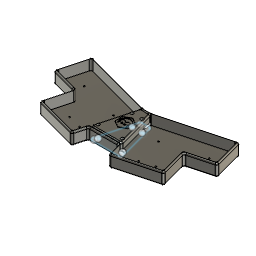
rattlemebonez32 v7 (Autodesk Fusion 360 design; units mm, degrees)
Autodesk Fusion 360 part; units mm, degrees
sketch "complete_combo(6)" plane through (0, 0, 0) normal (0, 0, 1) x (1, 0, 0)
  line L0 (-3.352867, 24.192112) -> (4.411704, 53.169887)
  line L1 (6.861194, 54.5841) -> (80.98315, 34.723182)
  line L2 (81.500788, 34.655034) -> (87.939454, 34.655034)
  line L3 (88.457092, 34.723182) -> (162.579048, 54.5841)
  line L4 (165.028537, 53.169887) -> (172.793109, 24.192112)
  line L5 (171.378895, 21.742622) -> (146.264824, 15.013327)
  line L6 (144.85061, 12.563837) -> (151.579905, -12.550234)
  line L7 (150.165692, -14.999724) -> (106.699029, -26.646581)
  line L8 (104.24954, -25.232367) -> (101.28209, -14.157694)
  line L9 (99.350238, -12.675332) -> (70.090004, -12.675332)
  line L10 (68.158152, -14.157694) -> (65.190702, -25.232367)
  line L11 (62.741212, -26.646581) -> (19.27455, -14.999724)
  line L12 (17.860337, -12.550234) -> (24.589632, 12.563837)
  line L13 (23.175418, 15.013327) -> (-1.938653, 21.742622)
  arc A0 (6.861194, 54.5841) -> (4.411705, 53.169887) centre (6.343556, 52.652249) ccw
  arc A1 (80.98315, 34.723182) -> (81.500788, 34.655034) centre (81.500788, 36.655034) ccw
  arc A2 (87.939454, 34.655034) -> (88.457092, 34.723182) centre (87.939454, 36.655034) ccw
  arc A3 (165.028537, 53.169887) -> (162.579048, 54.5841) centre (163.096686, 52.652249) ccw
  arc A4 (171.378895, 21.742622) -> (172.793109, 24.192112) centre (170.861257, 23.674474) ccw
  arc A5 (146.264824, 15.013327) -> (144.85061, 12.563837) centre (146.782462, 13.081475) ccw
  arc A6 (150.165692, -14.999724) -> (151.579905, -12.550234) centre (149.648054, -13.067872) ccw
  arc A7 (104.24954, -25.232367) -> (106.699029, -26.646581) centre (106.181391, -24.714729) ccw
  arc A8 (101.28209, -14.157694) -> (99.350238, -12.675332) centre (99.350238, -14.675332) ccw
  arc A9 (70.090004, -12.675332) -> (68.158152, -14.157694) centre (70.090004, -14.675332) ccw
  arc A10 (62.741212, -26.646581) -> (65.190702, -25.232367) centre (63.25885, -24.714729) ccw
  arc A11 (17.860337, -12.550234) -> (19.27455, -14.999724) centre (19.792188, -13.067872) ccw
  arc A12 (24.589632, 12.563837) -> (23.175418, 15.013327) centre (22.65778, 13.081475) ccw
  arc A13 (-3.352867, 24.192112) -> (-1.938653, 21.742622) centre (-1.421015, 23.674474) ccw
  line L14 (-1.51575, 25.252772) -> (5.472365, 51.332769)
  line L15 (7.921854, 52.746983) -> (79.146033, 33.662522)
  line L16 (79.663671, 33.594374) -> (89.776571, 33.594374)
  line L17 (90.294209, 33.662522) -> (161.518387, 52.746983)
  line L18 (163.967877, 51.332769) -> (170.955991, 25.252772)
  line L19 (169.541778, 22.803283) -> (144.427706, 16.073987)
  line L20 (143.013493, 13.624498) -> (149.742788, -11.489574)
  line L21 (148.328574, -13.939064) -> (107.75969, -24.809464)
  line L22 (105.3102, -23.39525) -> (102.34275, -12.320576)
  line L23 (100.410898, -10.838214) -> (69.029344, -10.838214)
  line L24 (67.097492, -12.320576) -> (64.130042, -23.39525)
  line L25 (61.680552, -24.809464) -> (21.111668, -13.939064)
  line L26 (19.697454, -11.489574) -> (26.426749, 13.624498)
  line L27 (25.012535, 16.073987) -> (-0.101536, 22.803283)
  arc A14 (7.921854, 52.746983) -> (5.472365, 51.332769) centre (7.404216, 50.815131) ccw
  arc A15 (79.146033, 33.662522) -> (79.663671, 33.594374) centre (79.663671, 35.594374) ccw
  arc A16 (89.776571, 33.594374) -> (90.294209, 33.662522) centre (89.776571, 35.594374) ccw
  arc A17 (163.967877, 51.332769) -> (161.518387, 52.746983) centre (162.036025, 50.815131) ccw
  arc A18 (169.541778, 22.803283) -> (170.955991, 25.252772) centre (169.02414, 24.735134) ccw
  arc A19 (144.427706, 16.073987) -> (143.013493, 13.624498) centre (144.945345, 14.142136) ccw
  arc A20 (148.328574, -13.939064) -> (149.742788, -11.489574) centre (147.810936, -12.007212) ccw
  arc A21 (105.3102, -23.39525) -> (107.75969, -24.809464) centre (107.242052, -22.877612) ccw
  arc A22 (102.34275, -12.320576) -> (100.410898, -10.838214) centre (100.410898, -12.838214) ccw
  arc A23 (69.029344, -10.838214) -> (67.097492, -12.320576) centre (69.029344, -12.838214) ccw
  arc A24 (61.680552, -24.809464) -> (64.130042, -23.39525) centre (62.19819, -22.877612) ccw
  arc A25 (19.697454, -11.489574) -> (21.111668, -13.939064) centre (21.629306, -12.007212) ccw
  arc A26 (26.426749, 13.624498) -> (25.012535, 16.073987) centre (24.494897, 14.142136) ccw
  arc A27 (-1.51575, 25.252772) -> (-0.101536, 22.803283) centre (0.416102, 24.735134) ccw
  line L28 (-0.903377, 25.606326) -> (5.825918, 50.720397)
  line L29 (8.275408, 52.134611) -> (78.53366, 33.308969)
  line L30 (79.051298, 33.24082) -> (90.388944, 33.24082)
  line L31 (90.906582, 33.308969) -> (161.164834, 52.134611)
  line L32 (163.614324, 50.720397) -> (170.343619, 25.606326)
  line L33 (143.815334, 16.427541) -> (168.929405, 23.156836)
  line L34 (142.40112, 13.978051) -> (149.130415, -11.136021)
  line L35 (108.113243, -24.197091) -> (147.716202, -13.58551)
  line L36 (102.696303, -11.708204) -> (105.663753, -22.782877)
  line L37 (100.764452, -10.225842) -> (68.67579, -10.225842)
  line L38 (63.776489, -22.782877) -> (66.743938, -11.708204)
  line L39 (21.72404, -13.58551) -> (61.326999, -24.197091)
  line L40 (20.309826, -11.136021) -> (27.039122, 13.978051)
  line L41 (0.510837, 23.156836) -> (25.624908, 16.427541)
  arc A28 (8.275408, 52.134611) -> (5.825918, 50.720397) centre (7.75777, 50.202759) ccw
  arc A29 (78.53366, 33.308969) -> (79.051298, 33.24082) centre (79.051298, 35.24082) ccw
  arc A30 (90.388944, 33.24082) -> (90.906582, 33.308969) centre (90.388944, 35.24082) ccw
  arc A31 (163.614324, 50.720397) -> (161.164834, 52.134611) centre (161.682472, 50.202759) ccw
  arc A32 (168.929405, 23.156836) -> (170.343619, 25.606325) centre (168.411767, 25.088687) ccw
  arc A33 (143.815334, 16.427541) -> (142.40112, 13.978051) centre (144.332972, 14.495689) ccw
  arc A34 (147.716202, -13.58551) -> (149.130415, -11.136021) centre (147.198564, -11.653659) ccw
  arc A35 (105.663753, -22.782877) -> (108.113243, -24.197091) centre (107.595605, -22.265239) ccw
  arc A36 (102.696303, -11.708204) -> (100.764452, -10.225842) centre (100.764452, -12.225842) ccw
  arc A37 (68.67579, -10.225842) -> (66.743939, -11.708204) centre (68.67579, -12.225842) ccw
  arc A38 (61.326999, -24.197091) -> (63.776489, -22.782877) centre (61.844637, -22.265239) ccw
  arc A39 (20.309826, -11.136021) -> (21.72404, -13.58551) centre (22.241678, -11.653659) ccw
  arc A40 (27.039122, 13.978051) -> (25.624908, 16.427541) centre (25.10727, 14.495689) ccw
  arc A41 (-0.903377, 25.606326) -> (0.510837, 23.156836) centre (1.028475, 25.088687) ccw
  circle A42 centre (16.950158, 34.281076) radius 2
  circle A43 centre (38.163361, -2.461271) radius 2
  circle A44 centre (52.652249, -6.343556) radius 2
  circle A45 centre (60.41682, 22.634219) radius 2
  circle A46 centre (152.490084, 34.281076) radius 2
  circle A47 centre (131.27688, -2.461271) radius 2
  circle A48 centre (116.787993, -6.343556) radius 2
  circle A49 centre (109.023422, 22.634219) radius 2
  circle A50 centre (16.950158, 34.281076) radius 0.8
  circle A51 centre (38.163361, -2.461271) radius 0.8
  circle A52 centre (52.652249, -6.343556) radius 0.8
  circle A53 centre (60.41682, 22.634219) radius 0.8
  circle A54 centre (152.490084, 34.281076) radius 0.8
  circle A55 centre (131.27688, -2.461271) radius 0.8
  circle A56 centre (116.787993, -6.343556) radius 0.8
  circle A57 centre (109.023422, 22.634219) radius 0.8
  circle A58 centre (71.591828, -5.206744) radius 2
  circle A59 centre (79.356399, 23.771031) radius 2
  circle A60 centre (97.848414, -5.206744) radius 2
  circle A61 centre (90.083843, 23.771031) radius 2
  circle A62 centre (71.591828, -5.206744) radius 0.8
  circle A63 centre (79.356399, 23.771031) radius 0.8
  circle A64 centre (97.848414, -5.206744) radius 0.8
  circle A65 centre (90.083843, 23.771031) radius 0.8
extrude "Extrude1" add sketch "complete_combo(6)" along normal blind 2 contours L14 L15 L16 L17 L18 L19 L20 L21 L22 L23 L24 L25 L26 L27 A14 A15 A16 A17 A18 A19 A20 A21 A22 A23 A24 A25 A26 A27 | L28 L29 L30 L31 L32 L33 L34 L35 L36 L37 L38 L39 L40 L41 A28 A29 A30 A31 A32 A33 A34 A35 A36 A37 A38 A39 A40 A41 | A42 | A43 | A44 | A45 | A46 | A47 | A48 | A49 | A58 | A59 | A60 | A61 | A62 | A63 | A64 | A65 picked at (79.489862, -10.429966) picked at (86.325586, 4.709558) picked at (18.539733, 34.14197) picked at (39.752937, -2.600377) picked at (54.244803, -6.442918) picked at (62.006396, 22.495113) picked at (151.815766, 32.83491) picked at (130.602562, -3.907436) picked at (115.528136, -7.32277) picked at (107.92358, 23.790268) picked at (70.33197, -6.185958) picked at (78.256558, 24.92708) picked at (96.588556, -6.185958) picked at (88.984001, 24.92708) picked at (71.787308, -4.945875) picked at (79.160919, 23.510162) picked at (98.043894, -4.945875) picked at (89.888362, 23.510162) makes body 1
extrude "Extrude2" add sketch "complete_combo(6)" along normal blind 13.1 contours L0 L1 L2 L3 L4 L5 L6 L7 L8 L9 L10 L11 L12 L13 A0 A1 A2 A3 A4 A5 A6 A7 A8 A9 A10 A11 A12 A13 picked at (79.843415, -11.450587) bodies 1
sketch "Sketch3" plane through (0, 0, 0) normal (0, 0, 1) x (1, 0, 0)
  line L0 (81.500788, 34.655034) -> (87.939454, 34.655034) construction
  line L1 (99.350238, -12.675332) -> (70.090004, -12.675332) construction
  line L2 (84.720121, 34.655034) -> (84.720121, -12.675332) construction
  line L3 (89.720121, 42.655034) -> (79.720121, 42.655034)
  line L4 (79.720121, 42.655034) -> (79.720121, 26.655034)
  line L5 (79.720121, 26.655034) -> (89.720121, 26.655034)
  line L6 (89.720121, 26.655034) -> (89.720121, 42.655034)
  line L7 (89.720121, 42.655034) -> (79.720121, 26.655034) construction
  line L8 (79.720121, 42.655034) -> (89.720121, 26.655034) construction
  point P0 (84.720121, 34.655034)
  dimension "d7" = 10
  dimension "d8" = 16
  constraint horizontal L3
  constraint perpendicular L3 L4
  constraint parallel L3 L5
  constraint parallel L4 L6
extrude "Extrude3" cut sketch "Sketch3" along normal blind 6 contours L3 L4 L5 L6 picked at (83.053454, 31.988367) bodies 1
sketch "center_combo" plane through (0, 0, 0) normal (0, 0, 1) x (1, 0, 0)
  line L0 (68.298698, -7.837613) -> (78.873758, 31.629049)
  line L1 (80.80561, 33.111411) -> (88.634632, 33.111411)
  line L2 (90.566484, 31.629049) -> (101.141544, -7.837613)
  line L3 (99.209692, -10.355251) -> (70.23055, -10.355251)
  arc A0 (80.80561, 33.111411) -> (78.873758, 31.629049) centre (80.80561, 31.111411) ccw
  arc A1 (90.566483, 31.629049) -> (88.634632, 33.111411) centre (88.634632, 31.111411) ccw
  arc A2 (99.209692, -10.355251) -> (101.141544, -7.837613) centre (99.209692, -8.355251) ccw
  arc A3 (68.298698, -7.837613) -> (70.23055, -10.355251) centre (70.23055, -8.355251) ccw
  circle A4 centre (71.591828, -5.206744) radius 0.8
  circle A5 centre (79.356399, 23.771031) radius 0.8
  circle A6 centre (97.848414, -5.206744) radius 0.8
  circle A7 centre (90.083843, 23.771031) radius 0.8
  circle A8 centre (71.591828, -5.206744) radius 1.65
  circle A9 centre (79.356399, 23.771031) radius 1.65
  circle A10 centre (90.083843, 23.771031) radius 1.65
  circle A11 centre (97.848414, -5.206744) radius 1.65
  dimension "d11" = 3.3
  dimension "d12" = 3.3
  dimension "d13" = 3.3
  dimension "d14" = 3.3
  constraint concentric A4 A8
  constraint concentric A5 A9
  constraint concentric A7 A10
  constraint concentric A6 A11
  measures "d11" diameter of A8
  measures "d12" diameter of A9
  measures "d13" diameter of A10
  measures "d14" diameter of A11
extrude "Extrude4" add sketch "center_combo" along normal blind 7.5 separate body contours L0 L1 L2 L3 A0 A1 A2 A3 picked at (86.307091, 4.688724) makes body 2
extrude "Extrude5" add sketch "center_combo" along normal blind 1 contours A8 | A9 | A10 | A11 picked at (70.982557, -3.987509) picked at (78.747128, 24.990265) picked at (88.913548, 24.469712) picked at (97.064231, -4.091934) bodies 2
move_body "Move1" bodies 2 to x (1, 0, 0) y (0, 1, 0) z (0, 0, 1) at (0, 0, 5.6)
fillet "Fillet1" radius 1.5 53 edges at (66.674427, -19.69503, 13.1) (68.872481, -13.088625, 13.1) (84.720121, -12.675332, 13.1) (100.567761, -13.088625, 13.1) (102.765815, -19.69503, 13.1) (105.181391, -26.44678, 13.1) (128.43236, -20.823152, 13.1) (151.380104, -14.067872, 13.1) (148.215258, 0.006802, 13.1) (145.050411, 14.081475, 13.1) (158.821859, 18.377975, 13.1) (172.593308, 22.674474, 13.1) (168.910823, 38.680999, 13.1) (164.096686, 54.384299, 13.1) (125.51807, 44.653641, 13.1) (88.200506, 34.672144, 13.1) (84.720121, 34.655034, 13.1) (81.239736, 34.672144, 13.1) (43.922172, 44.653641, 13.1) (5.343556, 54.384299, 13.1) (0.529419, 38.680999, 13.1) (-3.153066, 22.674474, 13.1) (10.618382, 18.377975, 13.1) (24.389831, 14.081475, 13.1) (21.224984, 0.006802, 13.1) (18.060138, -14.067872, 13.1) (41.007881, -20.823152, 13.1) (64.25885, -26.44678, 13.1) (126.149584, 44.822855, 0) (164.096686, 54.384299, 0) (168.910823, 38.680999, 0) (172.593308, 22.674474, 0) (158.821859, 18.377975, 0) (145.050411, 14.081475, 0) (148.215258, 0.006802, 0) (151.380104, -14.067872, 0) (128.43236, -20.823152, 0) (105.181391, -26.44678, 0) (102.765815, -19.69503, 0) (100.567761, -13.088625, 0) (84.720121, -12.675332, 0) (68.872481, -13.088625, 0) (66.674427, -19.69503, 0) (64.25885, -26.44678, 0) (41.007881, -20.823152, 0) (18.060138, -14.067872, 0) (21.224984, 0.006802, 0) (24.389831, 14.081475, 0) (10.618382, 18.377975, 0) (-3.153066, 22.674474, 0) (0.529419, 38.680999, 0) (5.343556, 54.384299, 0) (43.290658, 44.822855, 0) on bodies 1
sketch "Sketch5" plane through (0, 0, 13.1) normal (0, 0, 1) x (-1, 0, 0)
  circle A0 centre (-90.083843, -23.771031) radius 1.65
  circle A1 centre (-97.848414, 5.206744) radius 1.65
  circle A2 centre (-79.356399, -23.771031) radius 1.65
  circle A3 centre (-71.591828, 5.206744) radius 1.65
  arc A4 (-80.80561, -33.111411) -> (-78.873758, -31.629049) centre (-80.80561, -31.111411) ccw
  line L0 (-78.873758, -31.629049) -> (-68.298698, 7.837613)
  arc A5 (-68.298698, 7.837613) -> (-70.23055, 10.355251) centre (-70.23055, 8.355251) ccw
  line L1 (-70.23055, 10.355251) -> (-99.209692, 10.355251)
  arc A6 (-99.209692, 10.355251) -> (-101.141544, 7.837613) centre (-99.209692, 8.355251) ccw
  line L2 (-101.141544, 7.837613) -> (-90.566484, -31.629049)
  arc A7 (-90.566483, -31.629049) -> (-88.634632, -33.111411) centre (-88.634632, -31.111411) ccw
  line L3 (-88.634632, -33.111411) -> (-80.80561, -33.111411)
  spline S0 degree 3 poles (-80.077579, -10.893734) (-80.077579, -12.04043) (-81.008231, -12.971082) (-82.154927, -12.971082) knots 0 0 0 0 1 1 1 1
  spline S1 degree 3 poles (-82.154927, -12.971082) (-83.184569, -12.971082) (-84.040023, -12.220734) (-84.203943, -11.237384) knots 0 0 0 0 1 1 1 1
  spline S2 degree 3 poles (-84.203943, -11.237384) (-84.380777, -11.257897) (-84.560637, -11.268442) (-84.742944, -11.268442) knots 0 0 0 0 1 1 1 1
  spline S3 degree 3 poles (-84.742944, -11.268442) (-84.912928, -11.268442) (-85.080784, -11.259274) (-85.246044, -11.241407) knots 0 0 0 0 1 1 1 1
  spline S4 degree 3 poles (-85.246044, -11.241407) (-85.398464, -12.238228) (-86.260237, -13.002594) (-87.299452, -13.002594) knots 0 0 0 0 1 1 1 1
  spline S5 degree 3 poles (-87.299452, -13.002594) (-88.446149, -13.002594) (-89.376801, -12.071943) (-89.376801, -10.925246) knots 0 0 0 0 1 1 1 1
  spline S6 degree 3 poles (-89.376801, -10.925246) (-89.376801, -10.249874) (-89.053969, -9.649446) (-88.554305, -9.26996) knots 0 0 0 0 1 1 1 1
  spline S7 degree 3 poles (-88.554305, -9.26996) (-88.965566, -8.676582) (-89.241869, -7.982681) (-89.338691, -7.232783) knots 0 0 0 0 1 1 1 1
  spline S8 degree 3 poles (-89.338691, -7.232783) (-90.104795, -8.218124) (-90.561161, -9.456034) (-90.561161, -10.799887) knots 0 0 0 0 1 1 1 1
  spline S9 degree 3 poles (-90.561161, -10.799887) (-90.561161, -14.011542) (-87.954601, -16.618102) (-84.742946, -16.618102) knots 0 0 0 0 1 1 1 1
  spline S10 degree 3 poles (-84.742946, -16.618102) (-81.531291, -16.618102) (-78.924731, -14.011542) (-78.924731, -10.799887) knots 0 0 0 0 1 1 1 1
  spline S11 degree 3 poles (-78.924731, -10.799887) (-78.924731, -9.456035) (-79.381097, -8.218125) (-80.1472, -7.232784) knots 0 0 0 0 1 1 1 1
  spline S12 degree 3 poles (-80.1472, -7.232784) (-80.242047, -7.967386) (-80.509128, -8.64825) (-80.906588, -9.233523) knots 0 0 0 0 1 1 1 1
  spline S13 degree 3 poles (-80.906588, -9.233523) (-80.403219, -9.612727) (-80.077581, -10.215434) (-80.077579, -10.893734) knots 0 0 0 0 1 1 1 1
  spline S14 degree 3 poles (-84.104288, -9.042115) (-84.104219, -9.042115) (-84.104082, -9.042115) (-84.104014, -9.042115) knots 0 0 0 0 1 1 1 1
  spline S15 degree 3 poles (-84.104014, -9.042115) (-84.103977, -9.042115) (-83.786916, -9.042115) (-83.417422, -9.042115) knots 0 0 0 0 1 1 1 1
  spline S16 degree 3 poles (-83.417422, -9.042115) (-83.417422, -9.042138) (-83.417422, -9.728686) (-83.417422, -9.728708) knots 0 0 0 0 1 1 1 1
  spline S17 degree 3 poles (-83.417422, -9.728708) (-83.417422, -9.728731) (-83.417422, -9.737839) (-83.417422, -9.737862) knots 0 0 0 0 1 1 1 1
  line L4 (-83.417422, -9.737862) -> (-83.417216, -9.737862)
  spline S18 degree 3 poles (-83.417216, -9.737862) (-83.412415, -9.854624) (-83.316132, -9.947916) (-83.198196, -9.947916) knots 0 0 0 0 1 1 1 1
  spline S19 degree 3 poles (-83.198196, -9.947916) (-83.080259, -9.947916) (-82.98398, -9.854624) (-82.979176, -9.737862) knots 0 0 0 0 1 1 1 1
  line L5 (-82.979176, -9.737862) -> (-82.97897, -9.737862)
  spline S20 degree 3 poles (-82.97897, -9.737862) (-82.97897, -9.737724) (-82.97897, -9.728834) (-82.97897, -9.728708) knots 0 0 0 0 1 1 1 1
  spline S21 degree 3 poles (-82.97897, -9.728708) (-82.97897, -9.72857) (-82.97897, -9.042242) (-82.97897, -9.042116) knots 0 0 0 0 1 1 1 1
  spline S22 degree 3 poles (-82.97897, -9.042116) (-82.605575, -9.042116) (-82.283264, -9.042116) (-82.283226, -9.042116) knots 0 0 0 0 1 1 1 1
  line L6 (-82.283226, -9.042116) -> (-82.283226, -9.04191)
  spline S23 degree 3 poles (-82.283226, -9.04191) (-82.166463, -9.037108) (-82.073172, -8.940827) (-82.073172, -8.822891) knots 0 0 0 0 1 1 1 1
  spline S24 degree 3 poles (-82.073172, -8.822891) (-82.073172, -8.704955) (-82.166464, -8.608675) (-82.283226, -8.603872) knots 0 0 0 0 1 1 1 1
  line L7 (-82.283226, -8.603872) -> (-82.283226, -8.603667)
  line L8 (-82.283226, -8.603667) -> (-82.97897, -8.603667)
  spline S25 degree 3 poles (-82.97897, -8.603667) (-82.97897, -8.603601) (-82.97897, -7.917141) (-82.97897, -7.917075) knots 0 0 0 0 1 1 1 1
  spline S26 degree 3 poles (-82.97897, -7.917075) (-82.97897, -7.917009) (-82.97897, -7.907988) (-82.97897, -7.907922) knots 0 0 0 0 1 1 1 1
  line L9 (-82.97897, -7.907922) -> (-82.979176, -7.907922)
  spline S27 degree 3 poles (-82.979176, -7.907922) (-82.983978, -7.791159) (-83.080259, -7.697868) (-83.198195, -7.697868) knots 0 0 0 0 1 1 1 1
  spline S28 degree 3 poles (-83.198195, -7.697868) (-83.316131, -7.697868) (-83.412411, -7.791159) (-83.417214, -7.907922) knots 0 0 0 0 1 1 1 1
  line L10 (-83.417214, -7.907922) -> (-83.41742, -7.907922)
  spline S29 degree 3 poles (-83.41742, -7.907922) (-83.41742, -7.908059) (-83.41742, -7.916966) (-83.41742, -7.917075) knots 0 0 0 0 1 1 1 1
  spline S30 degree 3 poles (-83.41742, -7.917075) (-83.41742, -7.917212) (-83.41742, -8.603557) (-83.41742, -8.603667) knots 0 0 0 0 1 1 1 1
  spline S31 degree 3 poles (-83.41742, -8.603667) (-83.417489, -8.603667) (-84.103921, -8.603667) (-84.104011, -8.603667) knots 0 0 0 0 1 1 1 1
  spline S32 degree 3 poles (-84.104011, -8.603667) (-84.10408, -8.603667) (-84.113075, -8.603667) (-84.113165, -8.603667) knots 0 0 0 0 1 1 1 1
  line L11 (-84.113165, -8.603667) -> (-84.113165, -8.603872)
  spline S33 degree 3 poles (-84.113165, -8.603872) (-84.229928, -8.608674) (-84.32322, -8.704956) (-84.32322, -8.822892) knots 0 0 0 0 1 1 1 1
  spline S34 degree 3 poles (-84.32322, -8.822892) (-84.32322, -8.940829) (-84.229928, -9.037107) (-84.113165, -9.041911) knots 0 0 0 0 1 1 1 1
  line L12 (-84.113165, -9.041911) -> (-84.113165, -9.042117)
  line L13 (-84.113165, -9.042117) -> (-84.104288, -9.042115)
  spline S35 degree 3 poles (-86.773358, -9.618599) (-86.773295, -9.618535) (-86.773222, -9.618462) (-86.773153, -9.618394) knots 0 0 0 0 1 1 1 1
  spline S36 degree 3 poles (-86.773153, -9.618394) (-86.773127, -9.618368) (-86.548931, -9.394172) (-86.28766, -9.132901) knots 0 0 0 0 1 1 1 1
  spline S37 degree 3 poles (-86.28766, -9.132901) (-86.287644, -9.132917) (-85.802181, -9.618379) (-85.802165, -9.618395) knots 0 0 0 0 1 1 1 1
  spline S38 degree 3 poles (-85.802165, -9.618395) (-85.802149, -9.618411) (-85.795706, -9.624855) (-85.795692, -9.624868) knots 0 0 0 0 1 1 1 1
  line L14 (-85.795692, -9.624868) -> (-85.795555, -9.624731)
  spline S39 degree 3 poles (-85.795555, -9.624731) (-85.709594, -9.703898) (-85.575548, -9.701785) (-85.492154, -9.618388) knots 0 0 0 0 1 1 1 1
  spline S40 degree 3 poles (-85.492154, -9.618388) (-85.40876, -9.534994) (-85.406648, -9.400948) (-85.485811, -9.314987) knots 0 0 0 0 1 1 1 1
  line L15 (-85.485811, -9.314987) -> (-85.485674, -9.31485)
  spline S41 degree 3 poles (-85.485674, -9.31485) (-85.485743, -9.314782) (-85.492059, -9.308466) (-85.492147, -9.308377) knots 0 0 0 0 1 1 1 1
  spline S42 degree 3 poles (-85.492147, -9.308377) (-85.492216, -9.308308) (-85.977552, -8.822972) (-85.977641, -8.822883) knots 0 0 0 0 1 1 1 1
  spline S43 degree 3 poles (-85.977641, -8.822883) (-85.713611, -8.558853) (-85.485702, -8.330944) (-85.485675, -8.330917) knots 0 0 0 0 1 1 1 1
  line L16 (-85.485675, -8.330917) -> (-85.485812, -8.33078)
  spline S44 degree 3 poles (-85.485812, -8.33078) (-85.406644, -8.244819) (-85.408758, -8.110773) (-85.492149, -8.027379) knots 0 0 0 0 1 1 1 1
  spline S45 degree 3 poles (-85.492149, -8.027379) (-85.575542, -7.943986) (-85.709589, -7.941873) (-85.79555, -8.021043) knots 0 0 0 0 1 1 1 1
  line L17 (-85.79555, -8.021043) -> (-85.795686, -8.020906)
  line L18 (-85.795686, -8.020906) -> (-86.287652, -8.512872)
  spline S46 degree 3 poles (-86.287652, -8.512872) (-86.287699, -8.512825) (-86.773099, -8.027425) (-86.773146, -8.027378) knots 0 0 0 0 1 1 1 1
  spline S47 degree 3 poles (-86.773146, -8.027378) (-86.773192, -8.027331) (-86.779572, -8.020952) (-86.779619, -8.020904) knots 0 0 0 0 1 1 1 1
  line L19 (-86.779619, -8.020904) -> (-86.779756, -8.021042)
  spline S48 degree 3 poles (-86.779756, -8.021042) (-86.865717, -7.941874) (-86.999763, -7.943987) (-87.083157, -8.027378) knots 0 0 0 0 1 1 1 1
  spline S49 degree 3 poles (-87.083157, -8.027378) (-87.16655, -8.110771) (-87.168664, -8.244818) (-87.089493, -8.330779) knots 0 0 0 0 1 1 1 1
  line L20 (-87.089493, -8.330779) -> (-87.08963, -8.330916)
  spline S50 degree 3 poles (-87.08963, -8.330916) (-87.089562, -8.330984) (-87.083232, -8.337307) (-87.083157, -8.337389) knots 0 0 0 0 1 1 1 1
  spline S51 degree 3 poles (-87.083157, -8.337389) (-87.083089, -8.337458) (-86.597741, -8.822806) (-86.597663, -8.822883) knots 0 0 0 0 1 1 1 1
  spline S52 degree 3 poles (-86.597663, -8.822883) (-86.597727, -8.822947) (-87.083093, -9.308312) (-87.083156, -9.308376) knots 0 0 0 0 1 1 1 1
  spline S53 degree 3 poles (-87.083156, -9.308376) (-87.08322, -9.30844) (-87.089568, -9.314788) (-87.08963, -9.314849) knots 0 0 0 0 1 1 1 1
  line L21 (-87.08963, -9.314849) -> (-87.089493, -9.314987)
  spline S54 degree 3 poles (-87.089493, -9.314987) (-87.168659, -9.400947) (-87.166546, -9.534994) (-87.083156, -9.618387) knots 0 0 0 0 1 1 1 1
  spline S55 degree 3 poles (-87.083156, -9.618387) (-86.999762, -9.701781) (-86.865716, -9.703894) (-86.779755, -9.624731) knots 0 0 0 0 1 1 1 1
  line L22 (-86.779755, -9.624731) -> (-86.779619, -9.624868)
  line L23 (-86.779619, -9.624868) -> (-86.773358, -9.618599)
  line L24 (-91.735886, -14.962626) -> (-91.735889, -6.887865)
  line L25 (-91.735889, -6.887865) -> (-84.74294, -2.850488)
  line L26 (-84.74294, -2.850488) -> (-77.750002, -6.887863)
  line L27 (-77.750002, -6.887863) -> (-77.749999, -14.962622)
  line L28 (-77.749999, -14.962622) -> (-84.742948, -19)
  line L29 (-84.742948, -19) -> (-91.735886, -14.962626)
extrude "Extrude6" add sketch "Sketch5" along normal blind 0.5 contours L24 L25 L26 L27 L28 L29 picked at (-82.672529, -5.930941) bodies 2
fillet "Fillet2" radius 1.5 8 edges at (95.854014, 11.895718, 13.1) (89.852155, 32.698117, 13.1) (84.720121, 33.111411, 13.1) (79.588087, 32.698117, 13.1) (73.586228, 11.895718, 13.1) (68.643843, -9.572774, 13.1) (84.720121, -10.355251, 13.1) (100.796399, -9.572774, 13.1) on bodies 2
equation "floor_height = 2 mm"
equation "wall_height = center_plate_height + floor_height + STANDOFF_HEIGHT + PCB_THICKNESS"
equation "d3 = floor_height"
equation "d5 = wall_height"
equation "center_plate_height = 7.5 mm"
equation "STANDOFF_HEIGHT = 2 mm"
equation "PCB_THICKNESS = 1.6 mm"
equation "center_plate_screw_thickness = 1 mm"
equation "d19 = center_plate_height"
equation "d21 = center_plate_screw_thickness"
equation "case_outer_fillet = 1.5 mm"
equation "d25 = case_outer_fillet"
equation "d29 = case_outer_fillet"
